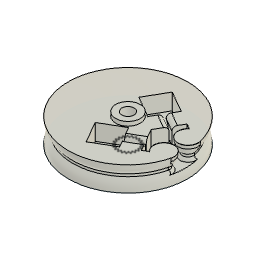
SG-90 Servo Motor_Filament Wheel v2 (Autodesk Fusion 360 design; units mm, degrees)
Autodesk Fusion 360 part; units mm, degrees
sketch "Main" plane through (0, 0, 28.3) normal (0, 0, 1) x (-1, 0, 0)
  arc A0 (2.75, -10.75) -> (-2.75, -10.75) centre (0, -10.75) ccw
  line L0 (-2.75, -10.75) -> (-2.75, -11.9144)
  arc A1 (-2.75, -11.9144) -> (2.75, -11.9144) centre (0, -16.85) ccw
  line L1 (2.75, -11.9144) -> (2.75, -10.75)
  line L2 (-2.4983, -16.8466) -> (-2.1166, -17.166)
  line L3 (-2.4983, -16.8466) -> (-2.1157, -16.5281)
  line L4 (-2.1157, -16.5281) -> (-2.3863, -16.1103)
  line L5 (-2.3863, -16.1103) -> (-1.9268, -15.9188)
  line L6 (-1.9268, -15.9188) -> (-2.0623, -15.4398)
  line L7 (-2.0623, -15.4398) -> (-1.5667, -15.3923)
  line L8 (-1.5667, -15.3923) -> (-1.555, -14.8946)
  line L9 (-1.555, -14.8946) -> (-1.0675, -14.9952)
  line L10 (-1.0675, -14.9952) -> (-0.9095, -14.5231)
  line L11 (-0.9095, -14.5231) -> (-0.4733, -14.763)
  line L12 (-0.4733, -14.763) -> (-0.1833, -14.3584)
  line L13 (-0.1833, -14.3584) -> (0.1629, -14.7162)
  line L14 (0.1629, -14.7162) -> (0.5593, -14.4151)
  line L15 (0.5593, -14.4151) -> (0.7846, -14.859)
  line L16 (0.7846, -14.859) -> (1.2521, -14.6881)
  line L17 (1.2521, -14.6881) -> (1.3366, -15.1787)
  line L18 (1.3366, -15.1787) -> (1.8337, -15.1532)
  line L19 (1.8337, -15.1532) -> (1.8337, -15.1532)
  line L20 (1.8337, -15.1532) -> (1.7698, -15.6469)
  line L21 (1.7698, -15.6469) -> (2.2524, -15.7691)
  line L22 (2.2524, -15.7691) -> (2.0458, -16.222)
  line L23 (2.0458, -16.222) -> (2.4709, -16.481)
  line L24 (2.4709, -16.481) -> (2.14, -16.8529)
  line L25 (2.14, -16.8529) -> (2.4699, -17.2258)
  line L26 (2.4699, -17.2258) -> (2.0441, -17.4836)
  line L27 (2.0441, -17.4836) -> (2.2494, -17.9371)
  line L28 (2.2494, -17.9371) -> (1.7665, -18.0579)
  line L29 (1.7665, -18.0579) -> (1.8291, -18.5518)
  line L30 (1.8291, -18.5518) -> (1.332, -18.525)
  line L31 (1.332, -18.525) -> (1.2462, -19.0153)
  line L32 (1.2462, -19.0153) -> (0.7791, -18.8432)
  line L33 (0.7791, -18.8432) -> (0.5526, -19.2864)
  line L34 (0.5526, -19.2864) -> (0.157, -18.9843)
  line L35 (0.157, -18.9843) -> (-0.1901, -19.3411)
  line L36 (-0.1901, -19.3411) -> (-0.4791, -18.9357)
  line L37 (-0.4791, -18.9357) -> (-0.9159, -19.1744)
  line L38 (-0.9159, -19.1744) -> (-1.0726, -18.7018)
  line L39 (-1.0726, -18.7018) -> (-1.5604, -18.8011)
  line L40 (-1.5604, -18.8011) -> (-1.5707, -18.3034)
  line L41 (-1.5707, -18.3034) -> (-2.0661, -18.2545)
  line L42 (-2.0661, -18.2545) -> (-1.9294, -17.7759)
  line L43 (-1.9294, -17.7759) -> (-2.3883, -17.5831)
  line L44 (-2.3883, -17.5831) -> (-2.1166, -17.166)
  circle A2 centre (0, -16.85) radius 14.625
  circle A3 centre (0, -16.85) radius 0.5
  dimension "d36" = 29.25
  dimension "d1" = 1
  constraint concentric A1 A2
  constraint concentric A2 A3
  measures "d36" diameter of A2
  measures "d1" diameter of A3
extrude "Extrude1" add sketch "Main" along normal blind 6 contours A0 L0 A1 L1 | A2
ref_plane "WorkPlane1" through (0, 16.85, 31.3) normal (0, 1, 0) x (0, 0, 1)
sketch "topLayout" plane through (0, 0, 34.3) normal (0, 0, 1) x (-1, 0, 0)
  circle A0 centre (0, -16.85) radius 1.5
  circle A1 centre (0, -16.85) radius 3
  circle A2 centre (0, -16.85) radius 14.625
  line L0 (0, -16.85) -> (-14.625, -16.85)
  line L1 (-14.625, -16.85) -> (0.6974, -25.6964) construction
  line L2 (-14.625, -16.85) -> (3.0678, -16.85) construction
  circle A3 centre (-11.7605, -19.8006) radius 2.5
  line L3 (-0.3, -27.4) -> (2.7, -22.2)
  line L4 (2.7, -22.2) -> (-2.4971, -19.2017)
  line L5 (-2.4971, -19.2017) -> (-5.4971, -24.4017)
  line L6 (-5.4971, -24.4017) -> (-0.3, -27.4)
  line L7 (-5.4971, -24.4017) -> (-10.1518, -21.7143)
  line L8 (-5.4971, -24.4017) -> (-10.8719, -24.4017) construction
  line L9 (-8.8971, -22.4387) -> (-5.6705, -16.85)
  line L10 (-7.2838, -19.6443) -> (-3.8847, -21.6068)
  line L11 (-7.5338, -20.0774) -> (-4.1346, -22.0399)
  line L12 (2.4699, -17.2258) -> (2.0441, -17.4836)
  line L13 (2.0441, -17.4836) -> (2.2494, -17.9371)
  line L14 (2.2494, -17.9371) -> (1.7665, -18.0579)
  line L15 (1.7665, -18.0579) -> (1.8291, -18.5518)
  line L16 (1.8291, -18.5518) -> (1.332, -18.525)
  line L17 (1.332, -18.525) -> (1.2462, -19.0153)
  line L18 (1.2462, -19.0153) -> (0.7791, -18.8432)
  line L19 (0.7791, -18.8432) -> (0.5526, -19.2864)
  line L20 (0.5526, -19.2864) -> (0.157, -18.9843)
  line L21 (0.157, -18.9843) -> (-0.1901, -19.3411)
  line L22 (-0.1901, -19.3411) -> (-0.4791, -18.9357)
  line L23 (-0.4791, -18.9357) -> (-0.9159, -19.1744)
  line L24 (-0.9159, -19.1744) -> (-1.0726, -18.7018)
  line L25 (-1.0726, -18.7018) -> (-1.5604, -18.8011)
  line L26 (-1.5604, -18.8011) -> (-1.5707, -18.3034)
  line L27 (-1.5707, -18.3034) -> (-2.0661, -18.2545)
  line L28 (-2.0661, -18.2545) -> (-1.9294, -17.7759)
  line L29 (-1.9294, -17.7759) -> (-2.3883, -17.5831)
  line L30 (-2.3883, -17.5831) -> (-2.1166, -17.166)
  line L31 (-2.1166, -17.166) -> (-2.4983, -16.8466)
  line L32 (-2.4983, -16.8466) -> (-2.1157, -16.5281)
  line L33 (-2.1157, -16.5281) -> (-2.3863, -16.1103)
  line L34 (-2.3863, -16.1103) -> (-1.9268, -15.9188)
  line L35 (-1.9268, -15.9188) -> (-2.0623, -15.4398)
  line L36 (-2.0623, -15.4398) -> (-1.5667, -15.3923)
  line L37 (-1.5667, -15.3923) -> (-1.555, -14.8946)
  line L38 (-1.555, -14.8946) -> (-1.0675, -14.9952)
  line L39 (-1.0675, -14.9952) -> (-0.9095, -14.5231)
  line L40 (-0.9095, -14.5231) -> (-0.4733, -14.763)
  line L41 (-0.4733, -14.763) -> (-0.1833, -14.3584)
  line L42 (-0.1833, -14.3584) -> (0.1629, -14.7162)
  line L43 (0.1629, -14.7162) -> (0.5593, -14.4151)
  line L44 (0.5593, -14.4151) -> (0.7846, -14.859)
  line L45 (0.7846, -14.859) -> (1.2521, -14.6881)
  line L46 (1.2521, -14.6881) -> (1.3366, -15.1787)
  line L47 (1.3366, -15.1787) -> (1.8337, -15.1532)
  line L48 (1.8337, -15.1532) -> (1.7698, -15.6469)
  line L49 (1.7698, -15.6469) -> (2.2524, -15.7691)
  line L50 (2.2524, -15.7691) -> (2.0458, -16.222)
  line L51 (2.0458, -16.222) -> (2.4709, -16.481)
  line L52 (2.4709, -16.481) -> (2.14, -16.8529)
  line L53 (2.14, -16.8529) -> (2.4699, -17.2258)
  dimension "d45" = 3
  dimension "d46" = 1.5
  dimension "d47" = 30
  dimension "d48" = 5
  dimension "d49" = 6
  dimension "d52" = 30
  dimension "d53" = 90
  dimension "d54" = 90
  constraint horizontal L0
  constraint coincident A2 L0.end
  constraint horizontal L2
  constraint tangent A2 A3
  constraint perpendicular L3 L4
  constraint parallel L3 L5
  constraint parallel L4 L6
  constraint horizontal L8
  constraint coincident A3 L7.end
  constraint coincident L7 L9.start
  constraint coincident L2 L9.end
  constraint midpoint L9 L10.start
  constraint coincident L5 L10.end
  constraint coincident L5 L11.end
  measures "d45" diameter of A0
  measures "d46" distance of A0
  measures "d47" angle of L1 L2
  measures "d48" diameter of A3
  measures "d49" distance of L3.start L5.end
  measures "d52" angle of L7 L8
  measures "d53" angle of L7 L9
  measures "d54" angle of L9 L10
sketch "outerChannel" plane through (0, 16.85, 0) normal (0, 1, 0) x (1, 0, 0)
  line L0 (-14.625, -34.3) -> (14.625, -34.3)
  line L1 (-14.625, -28.3) -> (14.625, -28.3)
  line L2 (0, -34.3) -> (0, -28.3)
  line L3 (0, -31.3) -> (-13.5, -31.3) construction
  line L4 (-14.625, -34.3) -> (-14.625, -28.3)
  line L5 (-13.5, -31.3) -> (-13.5, -31.6)
  line L6 (-13.5, -31.3) -> (-13.5, -31)
  spline S0 degree 5 poles (-14.625, -34.3) (-14.625, -34.1276) (-14.6157, -33.8066) (-14.5741, -33.3964) (-14.4676, -32.9681) (-14.2552, -32.5355) (-14.0131, -32.1971) (-13.7795, -31.9142) (-13.5975, -31.7077) (-13.5, -31.6) knots 0 0 0 0 0 0 0.2 0.4 0.6 0.8 1 1 1 1 1 1
  line L7 (-13.7417, -31.867) -> (-13.2583, -31.333)
  line L8 (-14.625, -34.7233) -> (-14.625, -33.8767)
  spline S1 degree 5 poles (-14.625, -28.3) (-14.625, -28.4724) (-14.6157, -28.7934) (-14.5741, -29.2036) (-14.4676, -29.6319) (-14.2552, -30.0645) (-14.0131, -30.4029) (-13.7795, -30.6858) (-13.5975, -30.8923) (-13.5, -31) knots 0 0 0 0 0 0 0.2 0.4 0.6 0.8 1 1 1 1 1 1
  line L9 (-14.625, -27.8767) -> (-14.625, -28.7233)
  line L10 (-13.7417, -30.733) -> (-13.2583, -31.267)
  dimension "d41" = 90
  dimension "d42" = 13.5
  dimension "d43" = 0.3
  constraint midpoint L0 L2.start
  constraint midpoint L1 L2.end
  constraint midpoint L2 L3.start
  constraint coincident L0.start L4.start
  constraint coincident L1.start L4.end
  constraint vertical L5
  constraint symmetric L5.start L3 L6.start
  constraint symmetric L3 L5.end L6.end
  constraint midpoint L5.end L7
  constraint midpoint L0.start L8
  constraint coincident L4 L8.end
  constraint symmetric L3 L0.start L1.start
  constraint symmetric L3 L7.start L10.start
  constraint symmetric L3 L7.end L10.end
  constraint symmetric L3 L8.start L9.start
  constraint symmetric L3 L8.end L9.end
  measures "d41" angle of L2 L3
  measures "d42" distance of L3.start L3.end
  measures "d43" distance of L3.end L5.end
revolve "Revolve1" cut sketch "outerChannel" angle 360 about axis through (0, 16.85, 28.3) along (0, 0, -1) contours L4 L5 L6 S0 L8 S1 L9
extrude "Extrude3" cut sketch "topLayout" against normal blind 4 contours A2 L0 A3 L7 L9 | L5 L9 L10 L11 | L3 L4 L5 L6
sketch "innerSphere" plane through (-6.438, 3.7142, 0) normal (-0.866186, 0.499722, 0) x (-0.499722, -0.866186, 0)
  line L0 (-21.1568, 34.3) -> (-23.8834, 34.3)
  line L1 (-23.8834, 34.3) -> (-23.8834, 30.3)
  line L2 (-23.8834, 30.3) -> (-21.1568, 30.3)
  line L3 (-21.1568, 30.3) -> (-21.1568, 34.3)
  line L4 (-20.6568, 34.3) -> (-20.6568, 30.3)
  line L5 (-20.6568, 30.3) -> (-21.1568, 30.3) construction
  line L6 (-20.9068, 30.3) -> (-20.9068, 33.3)
  circle A0 centre (-20.9068, 31.8) radius 1.5
  dimension "d60" = 90
  dimension "d61" = 3
  constraint coincident L4.end L5.start
  constraint coincident L2.end L3.start
  constraint midpoint L5 L6.start
  constraint midpoint L6 A0.centre
  constraint coincident L6.end A0
  measures "d60" angle of L5 L6
  measures "d61" distance of L6.start L6.end
revolve "Revolve2" cut sketch "innerSphere" angle 360 about axis through (4.0096, 21.8234, 30.3) along (0, 0, 1) contours L3 L6 A0 | L3 A0
ref_plane "WorkPlane2" through (0, 16.85, 31.3) normal (0.258819, -0.965926, 0) x (0, 0, 1)
ref_plane "WorkPlane3" through (11.7605, 19.8006, 32.3) normal (-0.258819, 0.965926, 0) x (0, 0, -1)
sketch "innerCurveChannel" plane through (-4.1624, 15.5341, 0) normal (-0.258819, 0.965926, 0) x (0, 0, -1)
  line L0 (-31.6, -17.4011) -> (-31.6, 9.1389)
  line L1 (-31.6, -17.8611) -> (-31.6, 8.6789)
  line L2 (-31.6, -17.6445) -> (-31, -17.6445)
  line L3 (-31, -17.8611) -> (-31, 8.6789)
  line L4 (-31.6, -17.8611) -> (-31, -17.8611)
  line L5 (-31, -17.8611) -> (-31, -19.8611)
  line L6 (-30.3, -19.8611) -> (-34.3, -19.8611)
  line L7 (-31.6, -19.8611) -> (-31.6, -17.8611)
  spline S0 degree 3 poles (-31, -17.6445) (-30.7886, -17.8594) (-30.5868, -18.0586) (-30.3562, -18.2605) (-30.3281, -18.2847) (-30.3, -18.3083) knots -0.109509 -0.109509 -0.109509 -0.109509 -0.01336 -0.01336 0 0 0 0
  line L8 (-30.3, -18.3083) -> (-30.3, -19.8611)
  spline S1 degree 3 poles (-34.3, -18.9842) (-34.2958, -18.9842) (-34.2915, -18.9841) (-33.9562, -18.9802) (-33.6421, -18.952) (-33.1099, -18.8152) (-32.8998, -18.7256) (-32.3869, -18.4077) (-32.0934, -18.1385) (-31.6916, -17.7373) (-31.6459, -17.6912) (-31.6, -17.6445) knots -0.434077 -0.434077 -0.434077 -0.434077 -0.432371 -0.432371 -0.296968 -0.296968 -0.185391 -0.185391 -0.020962 -0.020962 0 0 0 0
  line L9 (-31.6, -17.8611) -> (-31.6, 8.6789)
  spline S2 degree 5 poles (-34.3, 9.7656) (-34.1276, 9.7656) (-33.8066, 9.7566) (-33.3964, 9.7164) (-32.9681, 9.6135) (-32.5355, 9.4083) (-32.1971, 9.1745) (-31.9142, 8.9488) (-31.7077, 8.7731) (-31.6, 8.6789) knots 0 0 0 0 0 0 0.2 0.4 0.6 0.8 1 1 1 1 1 1
  line L10 (-34.3, 9.7656) -> (-34.3, -18.9861)
  spline S3 degree 5 poles (-34.3, -18.9861) (-34.1781, -18.9807) (-33.9359, -18.9653) (-33.5774, -18.9285) (-33.1098, -18.8498) (-32.5511, -18.6781) (-32.1377, -18.4451) (-31.856, -18.1896) (-31.6829, -17.9775) (-31.6, -17.8611) knots 0 0 0 0 0 0 0.2 0.4 0.6 0.8 1 1 1 1 1 1
  line L11 (-31.7965, -18.1371) -> (-31.4035, -17.5851)
  line L12 (-34.3, -18.9861) -> (-34.3, -19.8611)
  spline S4 degree 5 poles (-31, -17.8611) (-30.9713, -17.8895) (-30.9159, -17.944) (-30.8388, -18.0186) (-30.7447, -18.1063) (-30.6265, -18.2074) (-30.5163, -18.2905) (-30.4163, -18.3585) (-30.3403, -18.407) (-30.3, -18.4321) knots 0 0 0 0 0 0 0.2 0.4 0.6 0.8 1 1 1 1 1 1
  line L13 (-31.073, -17.7888) -> (-30.927, -17.9334)
  line L14 (-30.4024, -18.3684) -> (-30.1976, -18.4958)
  line L15 (-31, -17.4011) -> (-31.6, -17.4011)
  line L16 (-31, -17.4011) -> (-31, 9.1389)
  dimension "d65" = 0.6
  dimension "d66" = 2
  constraint horizontal L4
  constraint vertical L5
  constraint horizontal L6
  constraint vertical L7
  constraint coincident L1.start L4.start
  constraint vertical L8
  constraint coincident S0.end L8.start
  constraint coincident L5.end L6
  constraint coincident L10.end S3.start
  constraint midpoint L1.start L11
  constraint vertical L12
  constraint coincident L7.start L6
  constraint coincident L3.start L4.end
  constraint coincident L8 S4.end
  constraint midpoint L3.start L13
  constraint midpoint S4.end L14
  measures "d65" distance of L1.start L3.start
  measures "d66" distance of L1.start L7.start
revolve "Revolve3" cut sketch "innerCurveChannel" angle 230 about axis through (11.7605, 19.8006, 36.3) along (0, 0, -1) contours L4 L5 L6 L7 | L6 L7 S1 S3 L12 | L5 L6 L8 S4
fillet "Fillet1" radius 1 2 edges at (5.5842, 20.6256, 34.3) (5.8342, 21.0586, 34.3)
mirror "Mirror2" about plane through (0, 16.85, 31.3) normal (0, 1, 0) of "Extrude3", "Revolve2", "Revolve3", "Fillet1"
extrude "Extrude4" add sketch "topLayout" against normal blind 3 contours L12 L13 L14 L15 L16 L17 L18 L19 L20 L21 L22 L23 L24 L25 L26 L27 L28 L29 L30 L31 L32 L33 L34 L35 L36 L37 L38 L39 L40 L41 L42 L43 L44 L45 L46 L47 L48 L49 L50 L51 L52 L53
extrude "Extrude5" add sketch "topLayout" along normal blind 1 contours A1 | L12 L13 L14 L15 L16 L17 L18 L19 L20 L21 L22 L23 L24 L25 L26 L27 L28 L29 L30 L31 L32 L33 L34 L35 L36 L37 L38 L39 L40 L41 L42 L43 L44 L45 L46 L47 L48 L49 L50 L51 L52 L53
sketch "gearOffset" plane through (0, 0, 28.3) normal (0, 0, -1) x (1, 0, 0)
  line L0 (-2.4699, -17.2258) -> (-2.14, -16.8529)
  line L1 (-2.14, -16.8529) -> (-2.4709, -16.481)
  line L2 (-2.4709, -16.481) -> (-2.0458, -16.222)
  line L3 (-2.0458, -16.222) -> (-2.2524, -15.7691)
  line L4 (-2.2524, -15.7691) -> (-1.7698, -15.6469)
  line L5 (-1.7698, -15.6469) -> (-1.8337, -15.1532)
  line L6 (-1.8337, -15.1532) -> (-1.3366, -15.1787)
  line L7 (-1.3366, -15.1787) -> (-1.2521, -14.6881)
  line L8 (-1.2521, -14.6881) -> (-0.7846, -14.859)
  line L9 (-0.7846, -14.859) -> (-0.5593, -14.4151)
  line L10 (-0.5593, -14.4151) -> (-0.1629, -14.7162)
  line L11 (-0.1629, -14.7162) -> (0.1833, -14.3584)
  line L12 (0.1833, -14.3584) -> (0.4733, -14.763)
  line L13 (0.4733, -14.763) -> (0.9095, -14.5231)
  line L14 (0.9095, -14.5231) -> (1.0675, -14.9952)
  line L15 (1.0675, -14.9952) -> (1.555, -14.8946)
  line L16 (1.555, -14.8946) -> (1.5667, -15.3923)
  line L17 (1.5667, -15.3923) -> (2.0623, -15.4398)
  line L18 (2.0623, -15.4398) -> (1.9268, -15.9188)
  line L19 (1.9268, -15.9188) -> (2.3863, -16.1103)
  line L20 (2.3863, -16.1103) -> (2.1157, -16.5281)
  line L21 (2.1157, -16.5281) -> (2.4983, -16.8466)
  line L22 (2.4983, -16.8466) -> (2.1166, -17.166)
  line L23 (2.1166, -17.166) -> (2.3883, -17.5831)
  line L24 (2.3883, -17.5831) -> (1.9294, -17.7759)
  line L25 (1.9294, -17.7759) -> (2.0661, -18.2545)
  line L26 (2.0661, -18.2545) -> (1.5707, -18.3034)
  line L27 (1.5707, -18.3034) -> (1.5604, -18.8011)
  line L28 (1.5604, -18.8011) -> (1.0726, -18.7018)
  line L29 (1.0726, -18.7018) -> (0.9159, -19.1744)
  line L30 (0.9159, -19.1744) -> (0.4791, -18.9357)
  line L31 (0.4791, -18.9357) -> (0.1901, -19.3411)
  line L32 (0.1901, -19.3411) -> (-0.157, -18.9843)
  line L33 (-0.157, -18.9843) -> (-0.5526, -19.2864)
  line L34 (-0.5526, -19.2864) -> (-0.7791, -18.8432)
  line L35 (-0.7791, -18.8432) -> (-1.2462, -19.0153)
  line L36 (-1.2462, -19.0153) -> (-1.332, -18.525)
  line L37 (-1.332, -18.525) -> (-1.8291, -18.5518)
  line L38 (-1.8291, -18.5518) -> (-1.7665, -18.0579)
  line L39 (-1.7665, -18.0579) -> (-2.2494, -17.9371)
  line L40 (-2.2494, -17.9371) -> (-2.0441, -17.4836)
  line L41 (-2.0441, -17.4836) -> (-2.4699, -17.2258)
  circle A0 centre (0, -16.85) radius 14.625
  line L42 (1.6327, -14.7969) -> (1.645, -15.3194)
  line L43 (1.645, -15.3194) -> (2.1653, -15.3693)
  line L44 (2.1653, -15.3693) -> (2.0231, -15.8723)
  line L45 (2.0231, -15.8723) -> (2.5056, -16.0734)
  line L46 (2.5056, -16.0734) -> (2.2214, -16.5121)
  line L47 (2.2214, -16.5121) -> (2.6232, -16.8464)
  line L48 (2.6232, -16.8464) -> (2.2223, -17.1818)
  line L49 (2.2223, -17.1818) -> (2.5077, -17.6197)
  line L50 (2.5077, -17.6197) -> (2.0258, -17.8221)
  line L51 (2.0258, -17.8221) -> (2.1694, -18.3247)
  line L52 (2.1694, -18.3247) -> (1.6492, -18.3761)
  line L53 (1.6492, -18.3761) -> (1.6383, -18.8986)
  line L54 (1.6383, -18.8986) -> (1.1262, -18.7944)
  line L55 (1.1262, -18.7944) -> (0.9617, -19.2905)
  line L56 (0.9617, -19.2905) -> (0.503, -19.0399)
  line L57 (0.503, -19.0399) -> (0.1996, -19.4656)
  line L58 (0.1996, -19.4656) -> (-0.1648, -19.0909)
  line L59 (-0.1648, -19.0909) -> (-0.5802, -19.4082)
  line L60 (-0.5802, -19.4082) -> (-0.818, -18.9428)
  line L61 (-0.818, -18.9428) -> (-1.3085, -19.1235)
  line L62 (-1.3085, -19.1235) -> (-1.3985, -18.6087)
  line L63 (-1.3985, -18.6087) -> (-1.9205, -18.6369)
  line L64 (-1.9205, -18.6369) -> (-1.8548, -18.1183)
  line L65 (-1.8548, -18.1183) -> (-2.3618, -17.9914)
  line L66 (-2.3618, -17.9914) -> (-2.1462, -17.5153)
  line L67 (-2.1462, -17.5153) -> (-2.5933, -17.2445)
  line L68 (-2.5933, -17.2445) -> (-2.247, -16.8531)
  line L69 (-2.247, -16.8531) -> (-2.5944, -16.4626)
  line L70 (-2.5944, -16.4626) -> (-2.1481, -16.1906)
  line L71 (-2.1481, -16.1906) -> (-2.365, -15.7151)
  line L72 (-2.365, -15.7151) -> (-1.8583, -15.5868)
  line L73 (-1.8583, -15.5868) -> (-1.9254, -15.0684)
  line L74 (-1.9254, -15.0684) -> (-1.4034, -15.0952)
  line L75 (-1.4034, -15.0952) -> (-1.3147, -14.5801)
  line L76 (-1.3147, -14.5801) -> (-0.8238, -14.7595)
  line L77 (-0.8238, -14.7595) -> (-0.5872, -14.2934)
  line L78 (-0.5872, -14.2934) -> (-0.171, -14.6095)
  line L79 (-0.171, -14.6095) -> (0.1924, -14.2339)
  line L80 (0.1924, -14.2339) -> (0.497, -14.6587)
  line L81 (0.497, -14.6587) -> (0.955, -14.4068)
  line L82 (0.955, -14.4068) -> (1.1208, -14.9025)
  line L83 (1.1208, -14.9025) -> (1.6327, -14.7969)
extrude "Extrude6" cut sketch "gearOffset" against normal up to surface (3 mm away) contours L42 L43 L44 L45 L46 L47 L48 L49 L50 L51 L52 L53 L54 L55 L56 L57 L58 L59 L60 L61 L62 L63 L64 L65 L66 L67 L68 L69 L70 L71 L72 L73 L74 L75 L76 L77 L78 L79 L80 L81 L82 L83
equation "d36 = filamentWheel"
equation "filamentWheel = 29.25 mm"
equation "gearOffset = 0.08 mm"
equation "d3 = -gearOffset"
named bodies: "Filament Wheel"
